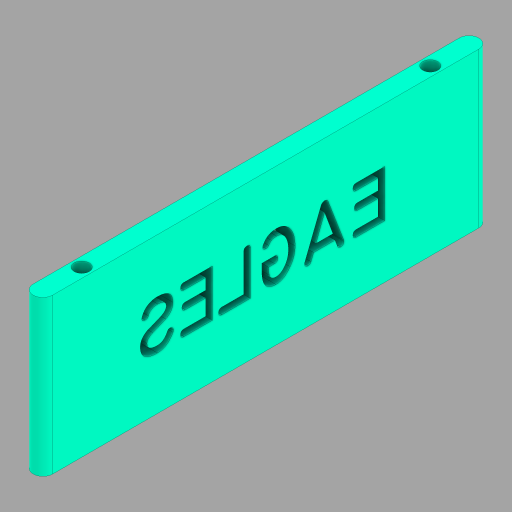
# Autodesk Inventor part: pod_akkum
Saved by Autodesk Inventor 2024.2 (Build 282272000, 272)
## iProperties
Created: 2024-02-02
Part Number: pod_akkum
Material: Типовые
Document SubType Name: Modeling
Designer: Fedor Orlov
Density: 1 g/cm^3
Appearance: По умолчанию
Author: Fedor Orlov
Autodesk Inventor part; units mm, degrees
ref_plane "YZ Plane" through (0, 0, 0) normal (1, 0, 0) x (0, 1, 0)
ref_plane "XZ Plane" through (0, 0, 0) normal (0, 1, 0) x (-1, 0, 0)
sketch "Эскиз12" plane through (0, 0, 0) normal (0, 1, 0) x (-1, 0, 0)
  line L0 (0, 45) -> (0, -45) construction
  circle A0 centre (0, 45) radius 1.5
  circle A1 centre (0, -45) radius 1.5
  line L1 (0, -55) -> (0, 55) construction
  line L2 (2.5, -55) -> (2.5, 55)
  line L3 (-2.5, 55) -> (-2.5, -55)
  arc A2 (-2.5, -55) -> (2.5, -55) centre (0, -55) ccw
  arc A3 (2.5, 55) -> (-2.5, 55) centre (0, 55) ccw
  point P0 (0, 0)
  point P1 (0, 0)
  dimension "d108" = 90
  dimension "d109" = 3
  dimension "d110" = 3
  dimension "d111" = 55
  dimension "d112" = 5
  constraints: 10 end point, 4 centre point, 4 point on circle, 4 tangent, 3 coincident, 2 midpoint, 2 vertical, 1 parallel
  measures "d108" distance of L0.start L0.end
  measures "d109" diameter of A0
  measures "d110" diameter of A1
  measures "d111" distance of point (0, 0) L1.end
  measures "d112" diameter of A3
extrude "Выдавливание12" add sketch "Эскиз12" along normal blind 40
sketch "Эскиз13" plane through (0, 40, 0) normal (0, 1, 0) x (1, 0, 0)
  circle A0 centre (0, -45) radius 1.5 projected
  circle A1 centre (0, -45) radius 1.95
  circle A2 centre (0, 45) radius 1.5 projected
  circle A3 centre (0, 45) radius 1.95
  point P0 (0, 0)
  dimension "d115" = 3.9
  dimension "d116" = 3.9
  constraints: 2 centre point, 2 coincident
  measures "d115" diameter of A1
  measures "d116" diameter of A3
extrude "Выдавливание13" cut sketch "Эскиз13" against normal blind 4 contours A0 | A1 | A2 | A3
ref_plane "РабПлоскость7" through (0, 20, 0) normal (0, 1, 0) x (1, 0, 0)
mirror "Зеркальное отражение3" about plane through (0, 20, 0) normal (0, 1, 0) of "Выдавливание13"
sketch "Эскиз14" plane through (-2.5, 0, -55) normal (-1, 0, 0) x (0, 0, 1)
  line L0 (55, 0) -> (55, 40)
  line L1 (110, 40) -> (0, 40) projected
  line L2 (22.9851, 26.2098) -> (87.0149, 26.2098) construction
  line L3 (87.0149, 26.2098) -> (87.0149, 13.7902) construction
  line L4 (87.0149, 13.7902) -> (22.9851, 13.7902) construction
  line L5 (22.9851, 13.7902) -> (22.9851, 26.2098) construction
  line L6 (22.9851, 26.2098) -> (87.0149, 13.7902) construction
  line L7 (31.5951, 13.768) -> (24.2585, 13.768)
  line L8 (24.2585, 13.768) -> (24.2585, 25.9055)
  line L9 (24.2585, 25.9055) -> (31.5951, 25.9055)
  spline S0 degree 2 poles (31.5951, 25.9055) (32.4742, 25.9055) (32.4742, 25.0603) knots 0 0 0 1 1 1
  spline S1 degree 2 poles (32.4742, 25.0603) (32.4742, 24.1925) (31.5951, 24.1925) knots 0 0 0 1 1 1
  line L10 (31.5951, 24.1925) -> (25.9715, 24.1925)
  line L11 (25.9715, 24.1925) -> (25.9715, 21.3413)
  line L12 (25.9715, 21.3413) -> (31.257, 21.3413)
  spline S2 degree 2 poles (31.257, 21.3413) (32.1135, 21.3413) (32.1135, 20.4735) knots 0 0 0 1 1 1
  spline S3 degree 2 poles (32.1135, 20.4735) (32.1135, 19.6057) (31.257, 19.6057) knots 0 0 0 1 1 1
  line L13 (31.257, 19.6057) -> (25.9715, 19.6057)
  line L14 (25.9715, 19.6057) -> (25.9715, 15.5036)
  line L15 (25.9715, 15.5036) -> (31.5951, 15.5036)
  spline S4 degree 2 poles (31.5951, 15.5036) (32.4742, 15.5036) (32.4742, 14.6358) knots 0 0 0 1 1 1
  spline S5 degree 2 poles (32.4742, 14.6358) (32.4742, 13.768) (31.5951, 13.768) knots 0 0 0 1 1 1
  spline S6 degree 2 poles (44.9159, 14.771) (44.9723, 14.602) (44.9723, 14.4442) knots 0 0 0 1 1 1
  spline S7 degree 2 poles (44.9723, 14.4442) (44.9723, 14.0723) (44.4088, 13.599) (44.0707, 13.599) knots 0 0 0 1 2 2 2
  spline S8 degree 2 poles (44.0707, 13.599) (43.4959, 13.599) (43.3044, 14.1399) knots 0 0 0 1 1 1
  line L16 (43.3044, 14.1399) -> (42.6056, 15.8417)
  line L17 (42.6056, 15.8417) -> (37.106, 15.8417)
  line L18 (37.106, 15.8417) -> (36.4636, 14.1512)
  spline S9 degree 2 poles (36.4636, 14.1512) (36.227, 13.599) (35.6522, 13.599) knots 0 0 0 1 1 1
  spline S10 degree 2 poles (35.6522, 13.599) (34.7845, 13.599) (34.7845, 14.4329) knots 0 0 0 1 1 1
  spline S11 degree 2 poles (34.7845, 14.4329) (34.7845, 14.5907) (34.8295, 14.726) knots 0 0 0 1 1 1
  line L19 (34.8295, 14.726) -> (38.9092, 25.4885)
  spline S12 degree 2 poles (38.9092, 25.4885) (39.2585, 26.0182) (39.7769, 26.0182) knots 0 0 0 1 1 1
  spline S13 degree 2 poles (39.7769, 26.0182) (40.2953, 26.0182) (40.656, 25.4998) knots 0 0 0 1 1 1
  line L20 (40.656, 25.4998) -> (44.9159, 14.771)
  line L21 (42.0309, 17.5547) -> (39.7995, 23.4262)
  line L22 (39.7995, 23.4262) -> (37.6357, 17.5547)
  line L23 (37.6357, 17.5547) -> (42.0309, 17.5547)
  spline S14 degree 2 poles (55.9828, 18.2308) (55.9828, 13.5539) (52.3539, 13.5539) knots 0 0 0 1 1 1
  spline S15 degree 2 poles (52.3539, 13.5539) (50.1676, 13.5539) (48.6913, 15.729) knots 0 0 0 1 1 1
  spline S16 degree 2 poles (48.6913, 15.729) (47.4065, 17.3743) (47.4065, 19.7072) knots 0 0 0 1 1 1
  spline S17 degree 2 poles (47.4065, 19.7072) (47.4065, 22.5584) (48.7814, 24.3052) knots 0 0 0 1 1 1
  spline S18 degree 2 poles (48.7814, 24.3052) (50.1338, 26.0182) (52.1624, 26.0182) knots 0 0 0 1 1 1
  spline S19 degree 2 poles (52.1624, 26.0182) (53.6387, 26.0182) (54.5741, 25.3533) knots 0 0 0 1 1 1
  spline S20 degree 2 poles (54.5741, 25.3533) (55.0023, 25.0603) (55.5658, 24.2038) knots 0 0 0 1 1 1
  spline S21 degree 2 poles (55.5658, 24.2038) (55.7574, 23.8882) (55.7574, 23.6403) knots 0 0 0 1 1 1
  spline S22 degree 2 poles (55.7574, 23.6403) (55.7574, 22.8401) (54.9347, 22.8401) knots 0 0 0 1 1 1
  spline S23 degree 2 poles (54.9347, 22.8401) (54.4839, 22.8401) (54.2247, 23.2233) knots 0 0 0 1 1 1
  spline S24 degree 2 poles (54.2247, 23.2233) (53.8077, 23.8093) (53.5035, 23.9897) knots 0 0 0 1 1 1
  spline S25 degree 2 poles (53.5035, 23.9897) (53.0414, 24.2827) (52.1624, 24.2827) knots 0 0 0 1 1 1
  spline S26 degree 2 poles (52.1624, 24.2827) (50.8213, 24.2827) (49.1308, 21.8146) (49.1308, 19.7184) knots 0 0 0 1 2 2 2
  spline S27 degree 2 poles (49.1308, 19.7184) (49.1308, 18.0167) (49.9197, 16.7996) knots 0 0 0 1 1 1
  spline S28 degree 2 poles (49.9197, 16.7996) (50.934, 15.2556) (52.3539, 15.2556) knots 0 0 0 1 1 1
  spline S29 degree 2 poles (52.3539, 15.2556) (53.6387, 15.2556) (54.0557, 16.484) knots 0 0 0 1 1 1
  spline S30 degree 2 poles (54.0557, 16.484) (54.236, 17.0362) (54.236, 18.3773) knots 0 0 0 1 1 1
  line L24 (54.236, 18.3773) -> (52.7146, 18.3773)
  spline S31 degree 2 poles (52.7146, 18.3773) (51.8693, 18.3773) (51.8693, 19.2451) knots 0 0 0 1 1 1
  spline S32 degree 2 poles (51.8693, 19.2451) (51.8693, 20.1129) (52.7146, 20.1129) knots 0 0 0 1 1 1
  line L25 (52.7146, 20.1129) -> (55.9828, 20.1129)
  line L26 (55.9828, 20.1129) -> (55.9828, 18.2308)
  line L27 (66.2833, 13.768) -> (58.9467, 13.768)
  line L28 (58.9467, 13.768) -> (58.9467, 25.0377)
  spline S33 degree 2 poles (58.9467, 25.0377) (58.9467, 25.9281) (59.8032, 25.9281) knots 0 0 0 1 1 1
  spline S34 degree 2 poles (59.8032, 25.9281) (60.6597, 25.9281) (60.6597, 25.0377) knots 0 0 0 1 1 1
  line L29 (60.6597, 25.0377) -> (60.6597, 15.5036)
  line L30 (60.6597, 15.5036) -> (66.2833, 15.5036)
  spline S35 degree 2 poles (66.2833, 15.5036) (67.1624, 15.5036) (67.1624, 14.6358) knots 0 0 0 1 1 1
  spline S36 degree 2 poles (67.1624, 14.6358) (67.1624, 13.768) (66.2833, 13.768) knots 0 0 0 1 1 1
  line L31 (76.0993, 13.768) -> (68.7627, 13.768)
  line L32 (68.7627, 13.768) -> (68.7627, 25.9055)
  line L33 (68.7627, 25.9055) -> (76.0993, 25.9055)
  spline S37 degree 2 poles (76.0993, 25.9055) (76.9783, 25.9055) (76.9783, 25.0603) knots 0 0 0 1 1 1
  spline S38 degree 2 poles (76.9783, 25.0603) (76.9783, 24.1925) (76.0993, 24.1925) knots 0 0 0 1 1 1
  line L34 (76.0993, 24.1925) -> (70.4757, 24.1925)
  line L35 (70.4757, 24.1925) -> (70.4757, 21.3413)
  line L36 (70.4757, 21.3413) -> (75.7612, 21.3413)
  spline S39 degree 2 poles (75.7612, 21.3413) (76.6177, 21.3413) (76.6177, 20.4735) knots 0 0 0 1 1 1
  spline S40 degree 2 poles (76.6177, 20.4735) (76.6177, 19.6057) (75.7612, 19.6057) knots 0 0 0 1 1 1
  line L37 (75.7612, 19.6057) -> (70.4757, 19.6057)
  line L38 (70.4757, 19.6057) -> (70.4757, 15.5036)
  line L39 (70.4757, 15.5036) -> (76.0993, 15.5036)
  spline S41 degree 2 poles (76.0993, 15.5036) (76.9783, 15.5036) (76.9783, 14.6358) knots 0 0 0 1 1 1
  spline S42 degree 2 poles (76.9783, 14.6358) (76.9783, 13.768) (76.0993, 13.768) knots 0 0 0 1 1 1
  spline S43 degree 2 poles (87.3802, 17.0701) (87.3802, 13.5314) (82.9512, 13.5314) knots 0 0 0 1 1 1
  spline S44 degree 2 poles (82.9512, 13.5314) (80.3705, 13.5314) (78.9167, 16.1572) knots 0 0 0 1 1 1
  spline S45 degree 2 poles (78.9167, 16.1572) (78.804, 16.3488) (78.804, 16.5855) knots 0 0 0 1 1 1
  spline S46 degree 2 poles (78.804, 16.5855) (78.804, 16.9686) (79.3675, 17.5321) (79.7394, 17.5321) knots 0 0 0 1 2 2 2
  spline S47 degree 2 poles (79.7394, 17.5321) (80.1789, 17.5321) (80.3817, 17.0926) knots 0 0 0 1 1 1
  spline S48 degree 2 poles (80.3817, 17.0926) (81.2157, 15.2444) (82.9512, 15.2444) knots 0 0 0 1 1 1
  spline S49 degree 2 poles (82.9512, 15.2444) (85.656, 15.2444) (85.656, 17.0362) knots 0 0 0 1 1 1
  spline S50 degree 2 poles (85.656, 17.0362) (85.656, 17.9942) (84.1346, 18.6929) knots 0 0 0 1 1 1
  spline S51 degree 2 poles (84.1346, 18.6929) (82.3201, 19.4254) (80.7875, 20.0453) knots 0 0 0 1 1 1
  spline S52 degree 2 poles (80.7875, 20.0453) (78.928, 21.1046) (78.928, 22.8627) knots 0 0 0 1 1 1
  spline S53 degree 2 poles (78.928, 22.8627) (78.928, 25.9844) (82.7484, 26.1422) knots 0 0 0 1 1 1
  spline S54 degree 2 poles (82.7484, 26.1422) (84.2135, 26.2098) (86.4787, 24.8574) (86.9182, 23.5276) knots 0 0 0 1 2 2 2
  spline S55 degree 2 poles (86.9182, 23.5276) (86.9858, 23.3811) (86.9858, 23.2459) knots 0 0 0 1 1 1
  spline S56 degree 2 poles (86.9858, 23.2459) (86.9858, 22.457) (86.0955, 22.457) knots 0 0 0 1 1 1
  spline S57 degree 2 poles (86.0955, 22.457) (85.4757, 22.457) (85.2841, 23.043) knots 0 0 0 1 1 1
  spline S58 degree 2 poles (85.2841, 23.043) (85.0587, 23.7079) (83.6725, 24.4743) (82.8273, 24.4292) knots 0 0 0 1 2 2 2
  spline S59 degree 2 poles (82.8273, 24.4292) (80.6748, 24.3278) (80.6748, 22.9078) knots 0 0 0 1 1 1
  spline S60 degree 2 poles (80.6748, 22.9078) (80.6748, 21.9048) (82.1736, 21.2398) knots 0 0 0 1 1 1
  spline S61 degree 2 poles (82.1736, 21.2398) (84.0219, 20.4622) (85.5207, 19.8988) knots 0 0 0 1 1 1
  spline S62 degree 2 poles (85.5207, 19.8988) (87.3802, 18.8619) (87.3802, 17.0701) knots 0 0 0 1 1 1
  point P0 (55, 20)
  constraints: 4 end point, 3 midpoint, 2 other
extrude "Выдавливание14" cut sketch "Эскиз14" against normal blind 5 contours S14 S15 S16 S17 S18 S19 S20 L0 S22 S23 S24 S25 S26 S27 S28 S29 S30 L24 S31 S32 L25 | L0 L25 L26 S14 | L0 S20 S21 S22 | L7 L8 L9 S0 S1 L10 L11 L12 S2 S3 L13 L14 L15 S4 S5 | S6 S7 S8 L16 L17 L18 S9 S10 S11 L19 S12 S13 L20 | L27 L28 S33 S34 L29 L30 S35 S36 | L31 L32 L33 S37 S38 L34 L35 L36 S39 S40 L37 L38 L39 S41 S42 | S43 S44 S45 S46 S47 S48 S49 S50 S51 S52 S53 S54 S55 S56 S57 S58 S59 S60 S61 S62
